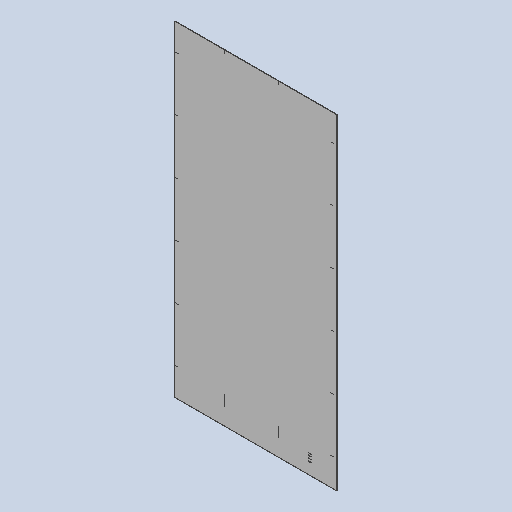
# Autodesk Inventor part: GBK 1325 shield 1.2
Saved by Autodesk Inventor 2026.2 (Build 302298000, 298)
## iProperties
Created: 2026-04-17
Part Number: GBK 1325 shield 1.2
Material: Steel
Document SubType Name: Sheet Metal
Designer: admin
Stock Number: 1325
Mass: 138487 g
Surface Area: 88564.8 cm^2
Volume: 17641.6 cm^3
Density: 7.85 g/cm^3
Flat Pattern Width: 148 cm
Flat Pattern Length: 298 cm
Flat Pattern Area: 44104 cm^2
Sheet Metal Rule: Default_mm
Sheet Metal Width: 1480,000 мм
Sheet Metal Length: 2980,000 мм
Sheet Metal Area: 4410400,000 мм^2
Appearance: Default
Project: 10
Author: admin
Autodesk Inventor part; units mm, degrees
ref_plane "YZ Plane" through (0, 0, 0) normal (1, 0, 0) x (0, 1, 0)
ref_plane "XZ Plane" through (0, 0, 0) normal (0, 1, 0) x (-1, 0, 0)
ref_plane "XY Plane" through (0, 0, 0) normal (0, 0, 1) x (1, 0, 0)
sketch "Sketch1" plane through (0, 0, 0) normal (0, 0, 1) x (1, 0, 0)
  line L0 (740, -1490) -> (-740, -1490)
  line L1 (-740, -1490) -> (-740, 1490)
  line L2 (-740, 1490) -> (740, 1490)
  line L3 (740, 1490) -> (740, -1490)
  line L4 (740, -1490) -> (-740, 1490) construction
  line L5 (-740, -1490) -> (740, 1490) construction
  point P0 (0, 0)
  dimension "d0" = 1480
  dimension "d1" = 2980
  measures "d0" distance of L1.end L2.end
  measures "d1" distance of L0.end L1.end
extrude "Plate2" add sketch "Sketch1" along normal blind 4
sketch "Sketch4" plane through (0, 0, 4) normal (0, 0, 1) x (1, 0, 0)
  line L0 (507.8568, -1305.8232) -> (507.8568, -1663.5137) construction
  line L1 (507.8568, -1663.5137) -> (476.5926, -1663.5137) construction
  line L2 (476.5926, -1663.5137) -> (476.5926, -1305.8232) construction
  line L3 (476.5926, -1305.8232) -> (507.8568, -1305.8232) construction
  line L4 (210.5058, -1238) -> (210.5058, -1335) projected
  line L5 (210.5058, -1335) -> (206.5068, -1335) projected
  line L6 (-289.6228, -1238) -> (-289.6228, -1335) projected
  line L7 (-289.6228, -1335) -> (-293.6218, -1335) projected
  ellipse E0 centre (210.5058, 1490.5) end of major axis (210.5058, 1520.5) minor radius 0.6803 (210.5058, 1460.5) -> (210.5058, 1520.5) ccw projected
  line L8 (210.5058, 1460.5) -> (206.5068, 1460.5) projected
  ellipse E1 centre (-289.6228, 1490.5) end of major axis (-289.6228, 1520.5) minor radius 0.6803 (-289.6228, 1460.5) -> (-289.6228, 1520.5) ccw projected
  line L9 (-289.6228, 1460.5) -> (-293.6218, 1460.5) projected
  line L10 (710, -1234.5) -> (710, -1230.5) projected
  line L11 (710, -737.8333) -> (710, -733.8333) projected
  line L12 (710, -241.1667) -> (710, -237.1667) projected
  line L13 (710, 255.5) -> (710, 259.5) projected
  line L14 (710, 752.1667) -> (710, 756.1667) projected
  line L15 (710, 1248.8333) -> (710, 1252.8333) projected
  line L16 (-739.3197, -1234.5) -> (-710, -1234.5) projected
  line L17 (-710, -1234.5) -> (-710, -1230.5) projected
  line L18 (-739.3197, -737.8333) -> (-710, -737.8333) projected
  line L19 (-710, -737.8333) -> (-710, -733.8333) projected
  line L20 (-739.3197, -241.1667) -> (-710, -241.1667) projected
  line L21 (-710, -241.1667) -> (-710, -237.1667) projected
  line L22 (-739.3197, 255.5) -> (-710, 255.5) projected
  line L23 (-710, 255.5) -> (-710, 259.5) projected
  line L24 (-739.3197, 752.1667) -> (-710, 752.1667) projected
  line L25 (-710, 752.1667) -> (-710, 756.1667) projected
  line L26 (-739.3197, 1248.8333) -> (-710, 1248.8333) projected
  line L27 (-710, 1248.8333) -> (-710, 1252.8333) projected
  line L28 (710, 1248.8333) -> (680, 1248.8333)
  line L29 (710, 752.1667) -> (680, 752.1667)
  line L30 (710, 255.5) -> (680, 255.5)
  line L31 (710, -241.1667) -> (680, -241.1667)
  line L32 (710, -737.8333) -> (680, -737.8333)
  line L33 (710, -1234.5) -> (680, -1234.5)
  point P0 (0, 0)
  dimension "d10" = 30
  dimension "d11" = 30
  dimension "d12" = 30
  dimension "d13" = 30
  dimension "d14" = 30
  dimension "d15" = 30
  constraints: 12 end point, 6 horizontal, 4 other
  measures "d10" distance of L15.start L28.end
  measures "d11" distance of L29.start L29.end
  measures "d12" distance of L30.start L30.end
  measures "d13" distance of L31.start L31.end
  measures "d14" distance of L32.start L32.end
  measures "d15" distance of L33.start L33.end
mark "Mark2"
equation "\"d0\" = Лист_ширина"
equation "\"d3\" = Thickness"
equation "\"BendRadius\" = Thickness"
equation "\"BendReliefWidth\" = Thickness"
equation "\"BendReliefDepth\" = 0.5 * Thickness"
equation "\"CornerReliefSize\" = 4 * Thickness"
equation "\"MinimumRemnant\" = 2 * Thickness"
equation "\"TransitionRadius\" = BendRadius"
equation "\"JacobiRadiusSize\" = BendRadius"
equation "\"GapSize\" = Thickness"
equation "\"Лист_ширина\" = 1480"
equation "\"Thickness\" = 4"
body "Solid2"
